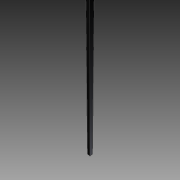
# Autodesk Inventor part: profil_handle
Saved by Autodesk Inventor 2015 (Build 190159000, 159)
## iProperties
Created: 2017-05-03
Part Number: profil_handle
Material: Generic
Document SubType Name: Modeling
Designer: miki
Density: 1 g/cm^3
Appearance: Glossy - Black
Author: miki
Autodesk Inventor part; units mm, degrees
ref_plane "YZ Plane" through (0, 0, 0) normal (1, 0, 0) x (0, 1, 0)
ref_plane "XZ Plane" through (0, 0, 0) normal (0, 1, 0) x (-1, 0, 0)
ref_plane "XY Plane" through (0, 0, 0) normal (0, 0, 1) x (1, 0, 0)
sketch "Sketch1" plane through (0, 0, 0) normal (0, 0, 1) x (1, 0, 0)
  line L0 (0, 0) -> (20, 0)
  line L1 (20, 0) -> (20, -20)
  line L2 (20, -20) -> (0, -20)
  line L3 (0, -20) -> (0, 0)
  dimension "d0" = 20
  dimension "d1" = 20
  constraints: 8 end point, 2 parallel, 1 horizontal, 1 perpendicular
  measures "d0" distance of L1.end L2.end
  measures "d1" distance of L0.end L1.end
extrude "Extrusion1" add sketch "Sketch1" along normal blind 850
sketch "Sketch2" plane through (0, 0, 850) normal (0, 0, 1) x (1, 0, 0)
  line L0 (1, -1) -> (19, -1)
  line L1 (19, -1) -> (19, -19)
  line L2 (19, -19) -> (1, -19)
  line L3 (1, -19) -> (1, -1)
  line L4 (0, 0) -> (0, -20) projected
  line L5 (20, 0) -> (0, 0) projected
  dimension "d4" = 1
  dimension "d5" = 1
  dimension "d6" = 18
  dimension "d7" = 18
  constraints: 8 end point, 2 parallel, 1 horizontal, 1 perpendicular
  measures "d4" distance between parallel lines of L4 L3
  measures "d5" distance between parallel lines of L5 L0
  measures "d6" distance of L0.end L1.end
  measures "d7" distance of L1.end L2.end
extrude "Extrusion2" cut sketch "Sketch2" against normal through all
body "Solid1"
